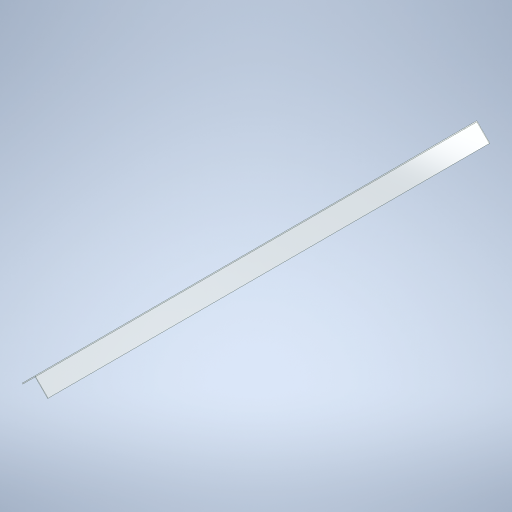
# Autodesk Inventor part: Shingles_On_Ridge_Vent
Saved by Autodesk Inventor 2024 (Build 280153000, 153)
## iProperties
Created: 2023-05-20
Part Number: Shingles_On_Ridge_Vent
Material: Steel
Document SubType Name: Modeling
Designer: Tom
Density: 7.85 g/cm^3
Appearance: Clear
Author: Tom
Autodesk Inventor part; units mm, degrees
ref_plane "YZ Plane" through (0, 0, 0) normal (1, 0, 0) x (0, 1, 0)
ref_plane "XZ Plane" through (0, 0, 0) normal (0, 1, 0) x (-1, 0, 0)
ref_plane "XY Plane" through (0, 0, 0) normal (0, 0, 1) x (1, 0, 0)
sketch "Sketch1" plane through (0, 0, 0) normal (0, 0, 1) x (1, 0, 0)
  line L0 (0, 0) -> (-224.5064, -224.5064)
  line L1 (-224.5064, -224.5064) -> (-215.5261, -233.4867)
  line L2 (-215.5261, -233.4867) -> (0, -17.9605)
  line L3 (0, -17.9605) -> (215.5261, -233.4867)
  line L4 (215.5261, -233.4867) -> (224.5064, -224.5064)
  line L5 (224.5064, -224.5064) -> (0, 0)
  line L6 (215.5261, -233.4867) -> (-215.5261, -233.4867)
  dimension "d0" = 12.7
  dimension "d4" = 304.8
  constraints: 14 end point, 7 perpendicular, 1 horizontal
  measures "d0" distance between parallel lines of L0 L2
  measures "d4" distance of L2.end L3.end
extrude "Extrusion1" add sketch "Sketch1" along normal blind 7620 contours L5 L4 L3 L2 L1 L0
body "Solid1"
